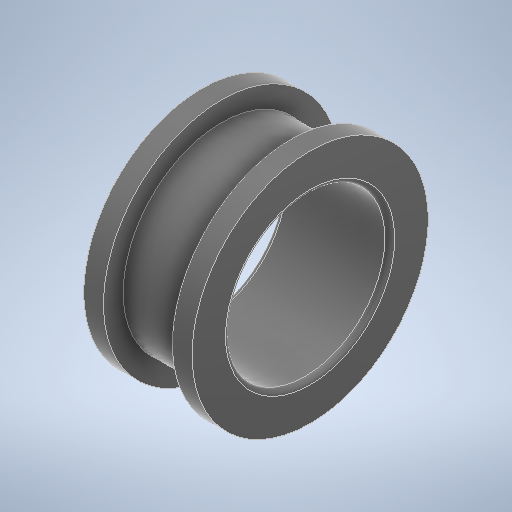
# Autodesk Inventor part: Idler_Pulley_Overlay
Saved by Autodesk Inventor 2025.1 (Build 291241020, 241B)
## iProperties
Created: 2024-11-07
Part Number: Idler_Pulley_Overlay
Material: ABS Plastic
Document SubType Name: Modeling
Designer: leon-
Density: 1.06 g/cm^3
Appearance: Smooth - Black
Author: leon-
Autodesk Inventor part; units mm, degrees
ref_plane "YZ Plane" through (0, 0, 0) normal (1, 0, 0) x (0, 1, 0)
ref_plane "XZ Plane" through (0, 0, 0) normal (0, 1, 0) x (-1, 0, 0)
ref_plane "XY Plane" through (0, 0, 0) normal (0, 0, 1) x (1, 0, 0)
sketch "Sketch1" plane through (0, 0, 0) normal (0, 0, 1) x (1, 0, 0)
  line L0 (5.5, 8.1) -> (5.5, 12)
  line L1 (5.5, 12) -> (3.5, 12)
  line L2 (3.5, 12) -> (3.5, 10)
  line L3 (3.5, 10) -> (0, 10)
  line L4 (5.5, 8.1) -> (0, 8.1)
  line L5 (0, 8.1) -> (0, 10)
  line L6 (-2.3, 0) -> (6.8, 0) projected
  line L7 (0, 5.6) -> (0, 23.1) projected
  line L8 (0, 14.6) -> (0, 8.1)
  line L9 (0, 20.6) -> (0, 14.6)
  point P0 (0, 9.05)
  point P1 (-1, 12)
  point P2 (4.5, 12)
  dimension "d0" = 5.5
  dimension "d1" = 3.5
  dimension "d2" = 10
  dimension "d3" = 12
  dimension "d4" = 8.1
  dimension "d8" = 1
  constraints: 16 end point, 4 perpendicular, 2 midpoint, 1 collinear, 1 horizontal, 1 vertical
  measures "d0" distance between parallel lines of L5 L0
  measures "d1" distance from line of point (0, 9.05) L2
  measures "d2" distance between parallel lines of L6 L3
  measures "d3" distance between parallel lines of L6 L1
  measures "d4" distance between parallel lines of L6 L4
  measures "d8" distance from line of L5 point (-1, 12)
revolve "Revolution1" add sketch "Sketch1" angle 360 about axis through (-10, 0, 0) along (1, 0, 0)
mirror "Mirror2" about plane through (0, 0, 0) normal (1, 0, 0) of "Revolution1"
fillet "Fillet1" radius 0.5 2 edges at (5.5, -8.1, 0) (-5.5, -8.1, 0)
body "Solid1"
